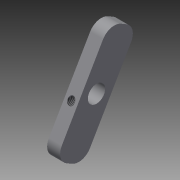
# Autodesk Inventor part: CAD:spring_arm
Saved by Autodesk Inventor 2015 (Build 190159000, 159)
## iProperties
Created: 2015-09-03
Material: Generic
Description: spring lever arm
Document SubType Name: Modeling
Designer: francis
Density: 1 g/cm^3
Appearance: Default
Mass: 6.2709 g
Surface Area: 32.5856 cm^2
Volume: 6.2709 cm^3
Part Category: insert part category here and press enter to fill value
Author: francis
Autodesk Inventor part; units mm, degrees
ref_plane "YZ Plane" through (0, 0, 0) normal (1, 0, 0) x (0, 1, 0)
ref_plane "XZ Plane" through (0, 0, 0) normal (0, 1, 0) x (-1, 0, 0)
ref_plane "XY Plane" through (0, 0, 0) normal (0, 0, 1) x (1, 0, 0)
sketch "Sketch1" plane through (0, 0, 0) normal (1, 0, 0) x (0, 1, 0)
  line L0 (1.0612, -13.162) -> (11.0434, 4.1278)
  line L1 (-1.0612, 13.162) -> (-11.0434, -4.1278)
  line L2 (6.0523, -4.5171) -> (-6.0523, 4.5171) construction
  line L3 (-26.5933, 0) -> (26.5933, 0) construction
  line L4 (0, -35.5609) -> (0, 35.5609) construction
  line L5 (11.0434, 4.1278) -> (18.9952, 17.9006)
  line L6 (18.9952, 17.9006) -> (6.0048, 25.4006)
  line L7 (-1.0612, 13.162) -> (6.0048, 25.4006)
  line L8 (1.0612, -13.162) -> (-6.0048, -25.4006)
  line L9 (-6.0048, -25.4006) -> (-18.9952, -17.9006)
  line L10 (-18.9952, -17.9006) -> (-11.0434, -4.1278)
  point P0 (0, 0)
  dimension "d1" = 15
  dimension "d2" = 50
  dimension "d4" = 60
  constraints: 18 end point, 4 point on line, 3 midpoint, 3 perpendicular, 2 parallel
  measures "d1" distance of L5.end L6.end
  measures "d2" distance of L8.end L5.end
  measures "d4" angle of L3 L1
extrude "Extrusion1" add sketch "Sketch1" along normal blind 6
sketch "Sketch2" plane through (0, 0, 0) normal (-1, 0, 0) x (0, 0, 1)
  point P0 (0, 0)
hole "Hole1" at (0, 0, 0) direction (1, 0, 0) diameter 8 end through all
sketch "Sketch3" plane through (0, 0, 0) normal (0, 1, 0) x (-1, 0, 0)
  line L0 (-6, -25.4006) -> (-6, 17.9006) construction
  line L1 (0, -25.4006) -> (0, 17.9006) construction
  line L2 (1.2, 0) -> (-7.2, 0) construction
  line L3 (0, 0) -> (-6, 0) construction
  point P0 (-6, -17.5083)
  point P1 (-6, 5.0083)
  point P2 (0, 5.0083)
  point P3 (0, -17.5083)
  point P4 (-3, 0)
  point P5 (-3, 0)
  constraints: 2 end point, 2 point on line, 1 coincident, 1 midpoint
hole "Hole2" at (3, 0, 0) direction (0, -1, 0) diameter 3.242 end through all thread size "M4x0.7" class "6H" standard "ISO Metric profile"
sketch "Sketch4" plane through (0, 0, 0) normal (-1, 0, 0) x (0, 0, 1)
  circle A0 centre (0, 0) radius 4 construction
  line L0 (-25.4006, -6.0048) -> (17.9006, 18.9952) construction
  line L1 (25.4006, 6.0048) -> (-17.9006, -18.9952) construction
  line L2 (-26.825, -15.4874) -> (32.6029, 18.8233) construction
  line L3 (7.5083, 12.9952) -> (-15.0083, -0.0048) construction
  line L4 (-17.9006, -18.9952) -> (-25.4006, -6.0048) projected
  line L5 (17.9006, 18.9952) -> (25.4006, 6.0048) projected
  point P0 (5.0083, 17.3253)
  point P1 (-17.5083, 4.3253)
  point P2 (17.3205, 10)
  point P3 (-17.3205, -10)
  dimension "d21" = 20
  dimension "d22" = 20
  constraints: 3 point on line, 2 end point, 1 parallel
  measures "d21" distance of point (0, 0) point (17.321, 10)
  measures "d22" distance of point (0, 0) point (-17.321, -10)
hole "Hole3" at (0, 10, 17.3205) at (0, -10, -17.3205) direction (1, 0, 0) diameter 3.459 depth 4 tip angle 118 thread size "M4x0.5" class "6H" standard "ISO Metric profile"
fillet "Fillet1" radius 6 4 edges at (3, 18.9952, 17.9006) (3, 6.0048, 25.4006) (3, -6.0048, -25.4006) (3, -18.9952, -17.9006)
body "Solid1"
